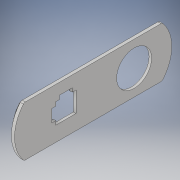
# Autodesk Inventor part: Controller top
Saved by Autodesk Inventor 2019 (Build 230136000, 136)
## iProperties
Created: 2019-05-05
Part Number: Controller top
Material: Generic
Document SubType Name: Modeling
Designer: Matthew XPS
Density: 1 g/cm^3
Appearance: Default
Author: Matthew XPS
Autodesk Inventor part; units mm, degrees
ref_plane "YZ Plane" through (0, 0, 0) normal (1, 0, 0) x (0, 1, 0)
ref_plane "XZ Plane" through (0, 0, 0) normal (0, 1, 0) x (-1, 0, 0)
ref_plane "XY Plane" through (0, 0, 0) normal (0, 0, 1) x (1, 0, 0)
sketch "Sketch1" plane through (0, 0, 0) normal (1, 0, 0) x (0, 1, 0)
  line L0 (-20, 55) -> (-20, -55)
  line L1 (-20, -55) -> (20, -55)
  line L2 (20, -55) -> (20, 55)
  line L3 (20, 55) -> (-20, 55)
  line L4 (-20, 55) -> (20, -55) construction
  line L5 (-20, -55) -> (20, 55) construction
  point P0 (0, 0)
  dimension "d0" = 110
  dimension "d1" = 40
  constraints: 12 end point, 2 midpoint, 2 parallel, 1 perpendicular, 1 vertical
  measures "d0" distance of L0.start L0.end
  measures "d1" distance of L1.end L0.end
extrude "Extrusion1" add sketch "Sketch1" along normal blind 2
sketch "Sketch2" plane through (2, 0, 0) normal (1, 0, 0) x (0, 0, -1)
  line L0 (55, 20) -> (-55, 20) projected
  line L1 (0, 20) -> (0, -25.4851) construction
  line L2 (-55, 20) -> (-55, -20) projected
  line L3 (-55, 0) -> (-48, 0)
  line L4 (-48, 0) -> (-48, 15)
  line L5 (-48, 15) -> (22, 15)
  line L6 (22, 15) -> (22, -15)
  line L7 (22, -15) -> (-48, -15)
  line L8 (-48, -15) -> (-48, 0)
  line L9 (-50.5, 12.5) -> (-45.5, 12.5)
  line L10 (-45.5, 12.5) -> (-45.5, 17.5)
  line L11 (-45.5, 17.5) -> (-50.5, 17.5)
  line L12 (-50.5, 17.5) -> (-50.5, 12.5)
  line L13 (-50.5, 12.5) -> (-45.5, 17.5) construction
  line L14 (-45.5, 12.5) -> (-50.5, 17.5) construction
  line L15 (-13, 15) -> (-13, -15)
  line L16 (24.5, 12.5) -> (19.5, 12.5)
  line L17 (19.5, 12.5) -> (19.5, 17.5)
  line L18 (19.5, 17.5) -> (24.5, 17.5)
  line L19 (24.5, 17.5) -> (24.5, 12.5)
  line L20 (24.5, 12.5) -> (19.5, 17.5) construction
  line L21 (19.5, 12.5) -> (24.5, 17.5) construction
  line L22 (-48, 0) -> (22, 0) construction
  line L23 (-50.5, -17.5) -> (-45.5, -17.5)
  line L24 (-45.5, -17.5) -> (-45.5, -12.5)
  line L25 (-45.5, -12.5) -> (-50.5, -12.5)
  line L26 (-50.5, -12.5) -> (-50.5, -17.5)
  line L27 (-50.5, -17.5) -> (-45.5, -12.5) construction
  line L28 (-45.5, -17.5) -> (-50.5, -12.5) construction
  line L29 (24.5, -17.5) -> (19.5, -17.5)
  line L30 (19.5, -17.5) -> (19.5, -12.5)
  line L31 (19.5, -12.5) -> (24.5, -12.5)
  line L32 (24.5, -12.5) -> (24.5, -17.5)
  line L33 (24.5, -17.5) -> (19.5, -12.5) construction
  line L34 (19.5, -17.5) -> (24.5, -12.5) construction
  point P0 (0, 0)
  dimension "d4" = 7
  dimension "d5" = 15
  dimension "d6" = 70
  dimension "d7" = 30
  dimension "d8" = 5
  dimension "d9" = 5
  dimension "d10" = 5
  dimension "d11" = 5
  dimension "d12" = 5
  dimension "d13" = 5
  constraints: 66 end point, 13 midpoint, 7 perpendicular, 6 parallel, 4 symmetric about line, 2 horizontal, 1 vertical
  measures "d4" distance of L3.start L3.end
  measures "d5" distance of L3.end L4.end
  measures "d6" distance of L4.end L5.end
  measures "d7" distance of L5.end L6.end
  measures "d8" distance of L9.start L9.end
  measures "d9" distance of L10.end L9.end
  measures "d10" distance of L23.start L23.end
  measures "d11" distance of L24.end L23.end
  measures "d12" distance of L29.start L29.end
  measures "d13" distance of L29.end L30.end
extrude "Extrusion2" add sketch "Sketch2" along normal blind 20
sketch "Sketch3" plane through (22, 0, 0) normal (1, 0, 0) x (0, 0, -1)
  line L0 (22, -12.5) -> (22, 12.5) projected
  line L1 (22, 12.5) -> (24.5, 12.5) projected
  line L2 (24.5, 12.5) -> (24.5, 17.5) projected
  line L3 (24.5, 17.5) -> (19.5, 17.5) projected
  line L4 (19.5, 17.5) -> (19.5, 15) projected
  line L5 (19.5, 15) -> (-45.5, 15) projected
  line L6 (-45.5, 15) -> (-45.5, 17.5) projected
  line L7 (-45.5, 17.5) -> (-50.5, 17.5) projected
  line L8 (-50.5, 17.5) -> (-50.5, 12.5) projected
  line L9 (-50.5, 12.5) -> (-48, 12.5) projected
  line L10 (-48, 12.5) -> (-48, -12.5) projected
  line L11 (-48, -12.5) -> (-50.5, -12.5) projected
  line L12 (-50.5, -12.5) -> (-50.5, -17.5) projected
  line L13 (-50.5, -17.5) -> (-45.5, -17.5) projected
  line L14 (-45.5, -17.5) -> (-45.5, -15) projected
  line L15 (-45.5, -15) -> (19.5, -15) projected
  line L16 (19.5, -15) -> (19.5, -17.5) projected
  line L17 (19.5, -17.5) -> (24.5, -17.5) projected
  line L18 (24.5, -17.5) -> (24.5, -12.5) projected
  line L19 (24.5, -12.5) -> (22, -12.5) projected
  line L20 (-13, 15) -> (-13, -15)
  line L21 (22, -15) -> (22, 15)
  line L22 (-48, 15) -> (-48, -15)
  line L23 (-48, -15) -> (22, 15) construction
  line L24 (22, -15) -> (-48, 15) construction
  line L25 (-38.7087, -2.3779) -> (12.7087, -2.3779)
  line L26 (12.7087, -2.3779) -> (12.7087, 2.3779)
  line L27 (12.7087, 2.3779) -> (-38.7087, 2.3779)
  line L28 (-38.7087, 2.3779) -> (-38.7087, -2.3779)
  line L29 (-38.7087, -2.3779) -> (12.7087, 2.3779) construction
  line L30 (12.7087, -2.3779) -> (-38.7087, 2.3779) construction
  line L31 (-10.5799, -13.0883) -> (-10.5799, 13.0883)
  line L32 (-10.5799, 13.0883) -> (-15.4201, 13.0883)
  line L33 (-15.4201, 13.0883) -> (-15.4201, -13.0883)
  line L34 (-15.4201, -13.0883) -> (-10.5799, -13.0883)
  line L35 (-10.5799, -13.0883) -> (-15.4201, 13.0883) construction
  line L36 (-10.5799, 13.0883) -> (-15.4201, -13.0883) construction
  line L37 (-45.5, 15) -> (-48, 15)
  line L38 (24.5, 17.5) -> (19.5, 17.5)
  line L39 (19.5, 17.5) -> (19.5, 15)
  line L40 (19.5, 15) -> (24.5, 15)
  line L41 (24.5, 15) -> (24.5, 17.5)
  line L42 (24.5, 12.5) -> (22, 12.5)
  line L43 (22, 12.5) -> (22, 17.5)
  line L44 (22, 17.5) -> (24.5, 17.5)
  line L45 (24.5, 17.5) -> (24.5, 12.5)
  line L46 (-48, 12.5) -> (-50.5, 12.5) projected
  line L47 (-50.5, 17.5) -> (-48, 17.5)
  line L48 (-48, 17.5) -> (-48, 12.5)
  line L49 (-48, 12.5) -> (-50.5, 12.5)
  line L50 (-50.5, 12.5) -> (-50.5, 17.5)
  line L51 (-50.5, 12.5) -> (-50.5, 17.5) projected
  line L52 (-50.5, 17.5) -> (-45.5, 17.5)
  line L53 (-45.5, 17.5) -> (-45.5, 15)
  line L54 (-45.5, 15) -> (-50.5, 15)
  line L55 (-50.5, 15) -> (-50.5, 17.5)
  line L56 (-50.5, -17.5) -> (-45.5, -17.5)
  line L57 (-45.5, -17.5) -> (-45.5, -15.0713)
  line L58 (-45.5, -15.0713) -> (-50.5, -15.0713)
  line L59 (-50.5, -15.0713) -> (-50.5, -17.5)
  line L60 (-45.5, -17.5) -> (-50.5, -17.5) projected
  line L61 (-50.5, -17.5) -> (-48, -17.5)
  line L62 (-48, -17.5) -> (-48, -12.5)
  line L63 (-48, -12.5) -> (-50.5, -12.5)
  line L64 (-50.5, -12.5) -> (-50.5, -17.5)
  line L65 (19.5, -17.5) -> (24.5, -17.5)
  line L66 (24.5, -17.5) -> (24.5, -15)
  line L67 (24.5, -15) -> (19.5, -15)
  line L68 (19.5, -15) -> (19.5, -17.5)
  line L69 (24.5, -12.5) -> (24.5, -17.5) projected
  line L70 (24.5, -17.5) -> (22, -17.5)
  line L71 (22, -17.5) -> (22, -12.5)
  line L72 (22, -12.5) -> (24.5, -12.5)
  line L73 (24.5, -12.5) -> (24.5, -17.5)
  point P0 (0, 0)
  point P1 (-13, 0)
  constraints: 100 end point, 21 parallel, 10 horizontal, 10 perpendicular, 9 midpoint, 1 point on line
extrude "Extrusion3" add sketch "Sketch3" along normal blind 9 contours L19 L18 L67 L21 | L21 L40 L2 L1 | L71 L17 L16 L67 | L67 L18 L17 L71 | L43 L3 L2 L40 | L40 L4 L3 L43 | L34 L33 L25 L20 | L20 L25 L31 L34 | L37 L48 L7 L6 | L32 L31 L27 L20 | L20 L27 L33 L32 | L14 L13 L62 L58 | L25 L33 L27 L20 | L20 L27 L31 L25 | L54 L8 L7 L48 | L22 L9 L8 L54 | L62 L13 L12 L58 | L58 L12 L11 L22 L62 | L25 L28 L27 L33 | L31 L27 L26 L25
sketch "Sketch4" plane through (31, 0, 0) normal (1, 0, 0) x (0, 0, -1)
  line L0 (-48, 15) -> (-45.5, 15) projected
  line L1 (-45.5, 15) -> (-45.5, 17.5) projected
  line L2 (-45.5, 17.5) -> (-50.5, 17.5) projected
  line L3 (-50.5, 17.5) -> (-50.5, 12.5) projected
  line L4 (-50.5, 12.5) -> (-48, 12.5) projected
  line L5 (-48, 12.5) -> (-48, 15) projected
  line L6 (-48, -15.0713) -> (-48, -12.5) projected
  line L7 (-48, -12.5) -> (-50.5, -12.5) projected
  line L8 (-50.5, -12.5) -> (-50.5, -17.5) projected
  line L9 (-50.5, -17.5) -> (-45.5, -17.5) projected
  line L10 (-45.5, -17.5) -> (-45.5, -15.0713) projected
  line L11 (-45.5, -15.0713) -> (-48, -15.0713) projected
  line L12 (22, -15) -> (19.5, -15) projected
  line L13 (19.5, -15) -> (19.5, -17.5) projected
  line L14 (19.5, -17.5) -> (24.5, -17.5) projected
  line L15 (24.5, -17.5) -> (24.5, -12.5) projected
  line L16 (24.5, -12.5) -> (22, -12.5) projected
  line L17 (22, -12.5) -> (22, -15) projected
  line L18 (22, 15) -> (22, 12.5) projected
  line L19 (22, 12.5) -> (24.5, 12.5) projected
  line L20 (24.5, 12.5) -> (24.5, 17.5) projected
  line L21 (24.5, 17.5) -> (19.5, 17.5) projected
  line L22 (19.5, 17.5) -> (19.5, 15) projected
  line L23 (19.5, 15) -> (22, 15) projected
  point P0 (0, 0)
extrude "Extrusion4" add sketch "Sketch4" along normal blind 3
sketch "Sketch5" plane through (22, 0, 0) normal (1, 0, 0) x (0, 0, -1)
  line L0 (-48, 15) -> (-48, 12.5) projected
  line L1 (-48, 12.5) -> (-48, -12.5) projected
  line L2 (-48, -12.5) -> (-48, -15.0713) projected
  line L3 (-48, -15.0713) -> (-45.5, -15.0713) projected
  line L4 (-45.5, -15.0713) -> (-45.5, -15) projected
  line L5 (-45.5, -15) -> (19.5, -15) projected
  line L6 (19.5, -15) -> (22, -15) projected
  line L7 (22, -15) -> (22, -12.5) projected
  line L8 (22, -12.5) -> (22, 12.5) projected
  line L9 (22, 12.5) -> (22, 15) projected
  line L10 (22, 15) -> (19.5, 15) projected
  line L11 (19.5, 15) -> (-45.5, 15) projected
  line L12 (-45.5, 15) -> (-48, 15) projected
  line L13 (12.7087, -2.3779) -> (-10.5799, -2.3779) projected
  line L14 (-10.5799, -2.3779) -> (-10.5799, -13.0883) projected
  line L15 (-10.5799, -13.0883) -> (-15.4201, -13.0883) projected
  line L16 (-15.4201, -13.0883) -> (-15.4201, -2.3779) projected
  line L17 (-15.4201, -2.3779) -> (-38.7087, -2.3779) projected
  line L18 (-38.7087, -2.3779) -> (-38.7087, 2.3779) projected
  line L19 (-38.7087, 2.3779) -> (-15.4201, 2.3779) projected
  line L20 (-15.4201, 2.3779) -> (-15.4201, 13.0883) projected
  line L21 (-15.4201, 13.0883) -> (-10.5799, 13.0883) projected
  line L22 (-10.5799, 13.0883) -> (-10.5799, 2.3779) projected
  line L23 (-10.5799, 2.3779) -> (12.7087, 2.3779) projected
  line L24 (12.7087, 2.3779) -> (12.7087, -2.3779) projected
  line L25 (-45.5, 15.1) -> (19.5, 15.1)
  line L26 (19.5, 15.1) -> (22.1, 15.1)
  line L27 (22.1, 15.1) -> (22.1, 12.5)
  line L28 (22.1, 12.5) -> (22.1, -12.5)
  line L29 (22.1, -12.5) -> (22.1, -15.1)
  line L30 (22.1, -15.1) -> (19.5, -15.1)
  line L31 (19.5, -15.1) -> (-45.4, -15.1)
  line L32 (-45.4, -15.1) -> (-45.4, -15.1713)
  line L33 (-45.4, -15.1713) -> (-48.1, -15.1713)
  line L34 (-48.1, -15.1713) -> (-48.1, -12.5)
  line L35 (-48.1, -12.5) -> (-48.1, 12.5)
  line L36 (-48.1, 12.5) -> (-48.1, 15.1)
  line L37 (-48.1, 15.1) -> (-45.5, 15.1)
  point P0 (0, 0)
  dimension "d20" = 0.1
  constraints: 26 end point, 12 other
  measures "d20" distance between parallel lines of L11 L25
extrude "Extrusion5" cut sketch "Sketch5" along normal blind 50 contours L25 L26 L27 L28 L29 L30 L31 L32 L33 L34 L35 L36 L37
sketch "Sketch7" plane through (31, 0, 0) normal (1, 0, 0) x (0, 0, -1)
  line L0 (12.7087, 2.3779) -> (-10.5799, 2.3779) projected
  line L1 (-10.5799, -2.3779) -> (12.7087, -2.3779) projected
  line L2 (-3.8945, 2.3779) -> (12.8589, 2.3779)
  line L3 (12.8589, 2.3779) -> (12.8589, -2.3779)
  line L4 (12.8589, -2.3779) -> (-3.8945, -2.3779)
  line L5 (-3.8945, -2.3779) -> (-3.8945, 2.3779)
  point P0 (0, 0)
  constraints: 8 end point, 2 parallel, 2 point on line, 1 horizontal, 1 perpendicular
extrude "Extrusion7" cut sketch "Sketch7" against normal blind 9
chamfer "Chamfer1" distance 9 angle 45 1 edges at (22, 0, -22)
sketch "Sketch9" plane through (2, 0, 0) normal (1, 0, 0) x (0, 0, -1)
  arc A0 (-55, 20) -> (-55, -20) centre (-32.6393, 0) ccw
  line L0 (-55, -20) -> (55, -20) projected
  line L1 (55, 20) -> (-55, 20) projected
  arc A1 (55, -20) -> (55, 20) centre (32.6393, 0) ccw
  arc A2 (-53.8996, 17.6) -> (-53.8996, -17.6) centre (-32.6393, 0) ccw
  line L2 (-53.8996, 17.6) -> (53.8996, 17.6)
  arc A3 (53.8996, -17.6) -> (53.8996, 17.6) centre (32.6393, 0) ccw
  line L3 (53.8996, -17.6) -> (-53.8996, -17.6)
  point P0 (0, 0)
  dimension "d34" = 30
  dimension "d35" = 30
  dimension "d36" = 2.4
  constraints: 8 point on circle, 4 centre point, 4 end point, 3 other
  measures "d34" radius of A0
  measures "d35" radius of A1
  measures "d36" radial gap between concentric circles of A0 A2
extrude "Extrusion8" add sketch "Sketch9" along normal blind 36
sketch "Sketch10" plane through (0, 0, 0) normal (-1, 0, 0) x (0, 0, 1)
  line L0 (55, -20) -> (-55, -20) projected
  line L1 (-55, 20) -> (55, 20) projected
  arc A0 (55, -20) -> (55, 20) centre (32.6393, 0) ccw projected
  arc A1 (-55, 20) -> (-55, -20) centre (-32.6393, 0) ccw projected
  point P0 (0, 0)
extrude "Extrusion9" add sketch "Sketch10" against normal blind 2
sketch "Sketch11" plane through (38, 0, 0) normal (1, 0, 0) x (0, 0, -1)
  line L0 (-53.8996, 17.6) -> (53.8996, 17.6) projected
  arc A0 (53.8996, -17.6) -> (53.8996, 17.6) centre (32.6393, 0) ccw projected
  line L1 (53.8996, -17.6) -> (-53.8996, -17.6) projected
  arc A1 (-53.8996, 17.6) -> (-53.8996, -17.6) centre (-32.6393, 0) ccw projected
  arc A2 (-55, 20) -> (-55, -20) centre (-32.6393, 0) ccw projected
  line L2 (-55, -20) -> (55, -20) projected
  arc A3 (55, -20) -> (55, 20) centre (32.6393, 0) ccw projected
  line L3 (55, 20) -> (-55, 20) projected
  line L4 (53.8619, 17.52) -> (-53.8619, 17.52)
  arc A4 (-53.8619, 17.52) -> (-53.8619, -17.52) centre (-32.6393, 0) ccw
  line L5 (-53.8619, -17.52) -> (53.8619, -17.52)
  arc A5 (53.8619, -17.52) -> (53.8619, 17.52) centre (32.6393, 0) ccw
  line L6 (-53.2888, 16.32) -> (53.2888, 16.32)
  arc A6 (53.2888, -16.32) -> (53.2888, 16.32) centre (32.6393, 0) ccw
  line L7 (53.2888, -16.32) -> (-53.2888, -16.32)
  arc A7 (-53.2888, 16.32) -> (-53.2888, -16.32) centre (-32.6393, 0) ccw
  point P0 (0, 0)
  dimension "d41" = 0.08
  dimension "d42" = 1.2
  constraints: 8 end point, 8 point on circle, 4 centre point, 6 other
  measures "d41" distance between parallel lines of L0 L4
  measures "d42" distance between parallel lines of L4 L6
extrude "Extrusion10" add sketch "Sketch11" against normal blind 2.5 separate body contours A5 L5 A4 L4
sketch "Sketch12" plane through (38, 0, 0) normal (1, 0, 0) x (0, 0, -1)
  line L0 (55, 20) -> (-55, 20) projected
  arc A0 (-55, 20) -> (-55, -20) centre (-32.6393, 0) ccw projected
  arc A1 (55, -20) -> (55, 20) centre (32.6393, 0) ccw projected
  line L1 (-55, -20) -> (55, -20) projected
  point P0 (0, 0)
extrude "Extrusion11" add sketch "Sketch12" along normal blind 2.5 bodies 2
sketch "Sketch13" plane through (22, 0, 0) normal (1, 0, 0) x (0, 0, -1)
  line L0 (-48, 12.5) -> (-48, -12.5) projected
  line L1 (-48, 0) -> (-29.8, 0)
  line L2 (-29.8, 0) -> (-32.8, 0)
  line L3 (-29.8, 0) -> (-29.8, 8.1)
  line L4 (-29.8, 8.1) -> (-13.6, 8.1)
  line L5 (-13.6, 8.1) -> (-13.6, -8.1)
  line L6 (-13.6, -8.1) -> (-29.8, -8.1)
  line L7 (-29.8, -8.1) -> (-29.8, 0)
  line L8 (-32.8, 0) -> (-32.8, 5)
  line L9 (-32.8, 5) -> (-29.8, 5)
  line L10 (-32.8, 0) -> (-32.8, -5)
  line L11 (-32.8, -5) -> (-29.8, -5)
  line L12 (-21.7, 8.1) -> (-21.7, 11.1)
  line L13 (-21.7, 11.1) -> (-16.7, 11.1)
  line L14 (-16.7, 11.1) -> (-16.7, 7.9077)
  line L15 (-21.7, 11.1) -> (-26.7, 11.1)
  line L16 (-26.7, 11.1) -> (-26.7, 7.9077)
  line L17 (-26.7, 11.1) -> (-16.7, 11.1)
  line L18 (-16.7, 11.1) -> (-16.7, 8.1)
  line L19 (-16.7, 8.1) -> (-26.7, 8.1)
  line L20 (-26.7, 8.1) -> (-26.7, 11.1)
  line L21 (-32.8, 5) -> (-29.8, 5)
  line L22 (-29.8, 5) -> (-29.8, -5)
  line L23 (-29.8, -5) -> (-32.8, -5)
  line L24 (-32.8, -5) -> (-32.8, 5)
  point P0 (0, 0)
  dimension "d47" = 18.2
  dimension "d48" = 3
  dimension "d50" = 8.1
  dimension "d51" = 16.2
  dimension "d52" = 16.2
  dimension "d53" = 5
  dimension "d54" = 5
  dimension "d55" = 3
  constraints: 48 end point, 8 perpendicular, 4 parallel, 4 point on line, 4 symmetric about line, 4 vertical, 3 horizontal, 2 midpoint, 1 collinear
  measures "d47" distance of L1.start L1.end
  measures "d48" distance of L1.end L2.end
  measures "d50" distance of L1.end L3.end
  measures "d51" distance of L3.end L4.end
  measures "d52" distance of L4.end L5.end
  measures "d53" distance of L2.end L8.end
  measures "d54" distance of L12.end L13.end
  measures "d55" distance of L12.start L12.end
extrude "Extrusion12" cut sketch "Sketch13" along normal blind 50 bodies 2
sketch "Sketch14" plane through (40.5, 0, 0) normal (1, 0, 0) x (0, 0, -1)
  arc A0 (55, -20) -> (55, 20) centre (32.6393, 0) ccw projected
  line L0 (0, 0) -> (55, 20)
  line L1 (55, 20) -> (55, 0)
  line L2 (55, 0) -> (0, 0)
  circle A1 centre (32.6393, 0) radius 13.95
  dimension "d58" = 27.9
  constraints: 6 end point, 1 centre point, 1 coincident, 1 perpendicular, 1 vertical
  measures "d58" diameter of A1
extrude "Extrusion13" cut sketch "Sketch14" against normal blind 50 contours A1 L0 | L0 A1 L2 | L2 A1 picked at (33.9931, 4.4486) bodies 2
sketch "Sketch15" plane through (40.5, 0, 0) normal (1, 0, 0) x (0, 0, -1)
  circle A0 centre (0, 0) radius 87.2959
  constraints: 1 centre point, 1 coincident
extrude "Extrusion14" cut sketch "Sketch15" against normal blind 50 bodies 1
fillet "Fillet3" radius 2 12 edges at (39.25, 20, 55) (39.25, 20, -55) (39.25, -20, -55) (39.25, -20, 55) (36.75, 17.52, 53.8619) (36.75, -17.52, 53.8619) (36.75, 16.32, 53.2888) (36.75, -16.32, 53.2888) (36.75, -17.52, -53.8619) (36.75, 17.52, -53.8619) (36.75, 16.32, -53.2888) (36.75, -16.32, -53.2888)
fillet "Fillet4" radius 0.5 16 edges at (35.5, -17.3134, -53.7829) (35.5, -17.52, 0) (35.5, -17.3134, 53.7829) (35.5, 0, 60.1593) (35.5, 17.3134, 53.7829) (35.5, 17.52, 0) (35.5, 17.3134, -53.7829) (35.5, 0, -60.1593) (35.5, 16.1026, -53.2032) (35.5, 16.32, 0) (35.5, 16.1026, 53.2032) (35.5, 0, 58.9593) (35.5, -16.1026, 53.2032) (35.5, -16.32, 0) (35.5, -16.1026, -53.2032) (35.5, 0, -58.9593)
fillet "Fillet5" radius 0.5 11 edges at (38, 9.6, 26.7) (38, 8.1, 28.25) (38, 6.55, 29.8) (38, 5, 31.3) (38, 0, 32.8) (38, -5, 31.3) (38, -8.1, 21.7) (38, 0, 13.6) (38, 8.1, 15.15) (38, 9.6, 16.7) (38, 11.1, 21.7)
fillet "Fillet6" radius 0.5 1 edges at (38, 0, -18.6893)
body "Solid1"
body "Solid2"
